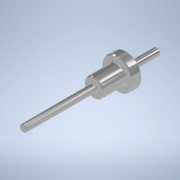
# Autodesk Inventor part: YTP-AP-E17-R1.0
Saved by Autodesk Inventor 2020.4 (Build 244396000, 396)
## iProperties
RuleStatus: InUse
AfterDocNew0: iPropertyEnforcement
BeforeDocSave0: Materialprüfung
Created: 2021-08-29
Part Number: YTP-AP-E17-R1.0
Material: Allgemein
Document SubType Name: Modeling
Designer: Uwe Wieser
Mass: 0.169249 g
Surface Area: 2.74041 cm^2
Volume: 0.169249 cm^3
Density: 1 g/cm^3
Appearance: Chrom - poliert
Project: Airbrush
Description: Ventilwelle
Werkstoff: 1.4301
Author: Uwe Wieser
Autodesk Inventor part; units mm, degrees
ref_plane "YZ Plane" through (0, 0, 0) normal (1, 0, 0) x (0, 1, 0)
ref_plane "XZ Plane" through (0, 0, 0) normal (0, 1, 0) x (-1, 0, 0)
ref_plane "XY Plane" through (0, 0, 0) normal (0, 0, 1) x (1, 0, 0)
sketch "Skizze1" plane through (0, 0, 0) normal (0, 0, 1) x (1, 0, 0)
  line L0 (-0.75, 28.5) -> (0, 28.5)
  line L1 (-3.3, 20) -> (-2, 20)
  line L2 (-2, 15) -> (-0.75, 15)
  line L3 (0, 28.5) -> (0, 0)
  line L4 (-0.75, 0) -> (-0.75, 15)
  line L5 (-2, 15) -> (-2, 20)
  line L6 (-3.3, 20) -> (-3.3, 22)
  line L7 (-0.75, 28.5) -> (-0.75, 22)
  line L8 (-0.75, 0) -> (0, 0)
  line L9 (-3.96, 0) -> (0.66, 0) projected
  line L10 (0, -5.7) -> (0, 34.2) projected
  line L11 (-0.75, 22) -> (-3.3, 22)
  point P0 (0, 0)
  dimension "d0" = 1.5
  dimension "d1" = 4
  dimension "d2" = 6.6
  dimension "d3" = 1.5
  dimension "d5" = 5
  dimension "d6" = 15
  dimension "d9" = 6.5
  dimension "d10" = 2
  constraints: 20 end point, 4 parallel, 2 horizontal, 2 point on line, 2 vertical
  measures "d0" diameter of L4 L10
  measures "d1" diameter of L5 L10
  measures "d2" diameter of L6 L10
  measures "d3" diameter of L7 L10
  measures "d5" distance between parallel lines of L2 L1
  measures "d6" distance between parallel lines of L9 L2
  measures "d9" distance from line of L6.end L0
  measures "d10" distance of L1.start L6.end
revolve "Umdrehung1" add sketch "Skizze1" angle 360 about axis through (0, -10, 0) along (0, 1, 0)
fillet "Rundung1" radius 0.2 3 edges at (0.75, 15, 0) (2, 20, 0) (0.75, 22, 0)
chamfer "Fase1" distance 0.2 angle 45 5 edges at (0.75, 0, 0) (2, 15, 0) (3.3, 20, 0) (3.3, 22, 0) (0.75, 28.5, 0)
